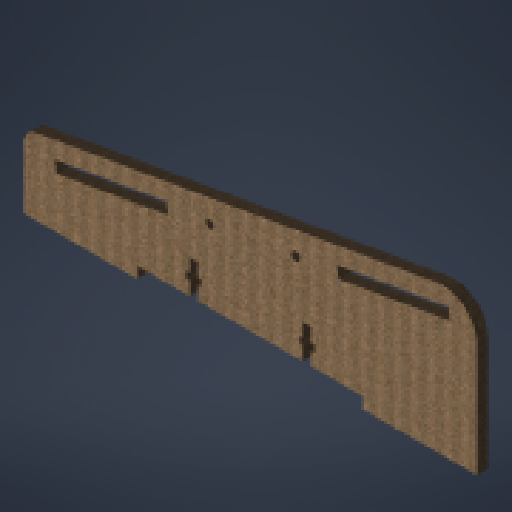
# Autodesk Inventor part: Pannel_Side
Saved by Autodesk Inventor 2024.1 (Build 281209000, 209)
## iProperties
Created: 2023-08-05
Part Number: Pannel_Side
Material: MDF Medium Density Fiberboard
Document SubType Name: Modeling
Designer: jaege
Density: 0.8 g/cm^3
Appearance: Cardboard - Corrugated
Author: jaege
Autodesk Inventor part; units mm, degrees
ref_plane "YZ Plane" through (0, 0, 0) normal (1, 0, 0) x (0, 1, 0)
ref_plane "XZ Plane" through (0, 0, 0) normal (0, 1, 0) x (-1, 0, 0)
ref_plane "XY Plane" through (0, 0, 0) normal (0, 0, 1) x (1, 0, 0)
sketch "Sketch1" plane through (0, 0, 0) normal (0, 0, 1) x (1, 0, 0)
  line L0 (0, 0) -> (40, 0) projected
  line L1 (40, 0) -> (40, 4) projected
  line L2 (0, 4) -> (40, 4) construction
  line L3 (0, 0) -> (0, 4) projected
  line L4 (120, 0) -> (160, 0) projected
  line L5 (160, 0) -> (160, 4) projected
  line L6 (120, 4) -> (160, 4) construction
  line L7 (120, 0) -> (120, 4) projected
  line L8 (0, 4) -> (0, 26.1116)
  line L9 (0, 26.1116) -> (160, 54.3239)
  line L10 (160, 54.3239) -> (160, 4)
  line L11 (120, 4) -> (101.5, 4)
  line L12 (61.5, 4) -> (61.5, 0) construction
  line L13 (58.5, 4) -> (58.5, 0) construction
  line L14 (98.5, 4) -> (98.5, 0) construction
  line L15 (101.5, 4) -> (101.5, 0) construction
  line L16 (58.5, 4) -> (61.5, 4) construction
  line L17 (61.5, 4) -> (61.5, 16)
  line L18 (61.5, 16) -> (58.5, 16)
  line L19 (58.5, 16) -> (58.5, 4)
  line L20 (57.3, 8.8) -> (62.7, 8.8)
  line L21 (62.7, 8.8) -> (62.7, 11.2)
  line L22 (62.7, 11.2) -> (57.3, 11.2)
  line L23 (57.3, 11.2) -> (57.3, 8.8)
  line L24 (98.5, 4) -> (101.5, 4) construction
  line L25 (101.5, 4) -> (101.5, 16)
  line L26 (101.5, 16) -> (98.5, 16)
  line L27 (98.5, 16) -> (98.5, 4)
  line L28 (102.7, 8.8) -> (97.3, 8.8)
  line L29 (97.3, 8.8) -> (97.3, 11.2)
  line L30 (97.3, 11.2) -> (102.7, 11.2)
  line L31 (102.7, 11.2) -> (102.7, 8.8)
  line L32 (58.5, 4) -> (40, 4)
  line L33 (61.5, 4) -> (58.5, 4)
  line L34 (98.5, 4) -> (61.5, 4)
  line L35 (101.5, 4) -> (98.5, 4)
  line L36 (11.5846, 18) -> (50.9769, 24.9459)
  line L37 (50.9769, 24.9459) -> (50.2823, 28.8852)
  line L38 (50.2823, 28.8852) -> (10.89, 21.9392)
  line L39 (10.89, 21.9392) -> (11.5846, 18)
  line L40 (110.7596, 39.5489) -> (150.1519, 46.4949)
  line L41 (150.1519, 46.4949) -> (150.8465, 42.5556)
  line L42 (150.8465, 42.5556) -> (111.4542, 35.6097)
  line L43 (111.4542, 35.6097) -> (110.7596, 39.5489)
  line L44 (150.1519, 46.4949) -> (160, 48.2314) construction
  line L45 (50.6296, 26.9155) -> (65.7489, 29.5815) construction
  line L46 (65.7489, 29.5815) -> (80.8682, 32.2474) construction
  line L47 (80.8682, 32.2474) -> (95.9876, 34.9134) construction
  line L48 (95.9876, 34.9134) -> (111.1069, 37.5793) construction
  circle A0 centre (65.7489, 29.5815) radius 1.5
  circle A1 centre (95.9876, 34.9134) radius 1.5
  point P0 (60, 11.2)
  point P1 (60, 16)
  point P2 (62.7, 10)
  point P3 (61.5, 10)
  point P4 (100, 11.2)
  point P5 (100, 16)
  point P6 (58.5, 8.8)
  point P7 (58.5, 11.2)
  point P8 (61.5, 11.2)
  point P9 (61.5, 8.8)
  point P10 (98.5, 8.8)
  point P11 (98.5, 11.2)
  point P12 (101.5, 11.2)
  point P13 (101.5, 8.8)
  dimension "d0" = 3
  dimension "d1" = 12
  dimension "d2" = 5.4
  dimension "d3" = 2.4
  dimension "d4" = 10
  dimension "d6" = 40
  dimension "d7" = 3
  dimension "d9" = 4
  dimension "d10" = 14
  dimension "d11" = 6
  dimension "d12" = 10
  dimension "d13" = 10
  constraints: 82 end point, 14 parallel, 11 perpendicular, 8 collinear, 8 midpoint, 5 vertical, 4 horizontal, 4 horizontal alignment, 4 point on line, 2 centre point, 2 coincident, 2 vertical alignment, 1 equal radius, 8 other
  measures "d0" distance of L18.end L17.end
  measures "d1" distance of L17.end L16.end
  measures "d2" distance of L21.end L22.end
  measures "d3" distance of L22.end L20.start
  measures "d4" distance from line of L8.end L39
  measures "d6" distance of L36.start L36.end
  measures "d7" diameter of A0
  measures "d9" distance between parallel lines of L36 L38
  measures "d10" distance from line of L2 L36.start
  measures "d11" distance between parallel lines of L9 L38
  measures "d12" distance of L40.end L44.end
  measures "d13" angle of L32 L36
extrude "Extrusion1" add sketch "Sketch1" along normal blind 4 contours L3 L8 L9 L10 L5 L4 L7 L11 L25 L28 L31 L30 L26 L27 L29 L34 L17 L20 L21 L22 L18 L19 L23 L32 L1 L0
fillet "Fillet1" radius 12 1 edges at (160, 54.3239, 2)
fillet "Fillet2" radius 5 1 edges at (0, 26.1116, 2)
body "Solid1"
